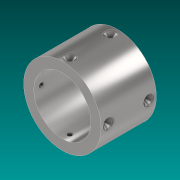
# Autodesk Inventor part: middenGearbox
Saved by Autodesk Inventor 2020.2 (Build 242310000, 310)
## iProperties
Created: 2020-05-14
Part Number: middenGearbox
Material: Stainless Steel
Document SubType Name: Modeling
Designer: Svend
Density: 8 g/cm^3
Appearance: Semi-Polished
Author: Svend
Autodesk Inventor part; units mm, degrees
ref_plane "XY Plane" through (0, 0, 0) normal (0, 0, 1) x (1, 0, 0)
sketch "Sketch1" plane through (0, 0, 0) normal (0, 0, 1) x (1, 0, 0)
  circle A0 centre (0, 0) radius 21
  circle A1 centre (0, 0) radius 15.5
  dimension "d0" = 42
  dimension "d1" = 31
  constraints: 2 centre point, 2 coincident
  measures "d0" diameter of A0
  measures "d1" diameter of A1
extrude "Extrusion1" add sketch "Sketch1" along normal mid plane 30
ref_plane "Work Plane1" through (21, 0, 0) normal (1, 0, 0) x (0, 1, 0)
ref_plane "Work Plane2" through (-21, 0, 0) normal (1, 0, 0) x (0, 1, 0)
ref_plane "Work Plane3" through (0, 21, 0) normal (0, 1, 0) x (-1, 0, 0)
ref_plane "Work Plane4" through (0, -21, 0) normal (0, 1, 0) x (-1, 0, 0)
sketch "Sketch3" plane through (-21, 0, 0) normal (1, 0, 0) x (0, 1, 0)
  line L0 (0, 21) -> (0, -21) projected
  line L1 (21, 15) -> (-21, 15) projected
  line L2 (-21, -15) -> (21, -15) projected
  point P0 (0, 0)
  point P1 (0, -11)
  point P2 (0, 11)
  dimension "d17" = 4
  dimension "d18" = 4
  constraints: 2 point on line
  measures "d17" distance from line of L2 point (0, -11)
  measures "d18" distance from line of L1 point (0, 11)
hole "Hole2" at (-21, 0, -11) at (-21, 0, 11) direction (1, 0, 0) diameter 6 depth 1
sketch "Sketch4" plane through (0, -21, 0) normal (0, 1, 0) x (-1, 0, 0)
  line L0 (21, 15) -> (-21, 15) projected
  line L1 (-21, -15) -> (21, -15) projected
  line L2 (0, -21) -> (0, 21) projected
  point P0 (0, 0)
  point P1 (0, -11)
  point P2 (0, 11)
  dimension "d26" = 4
  dimension "d27" = 4
  constraints: 2 point on line
  measures "d26" distance from line of L0 point (0, 11)
  measures "d27" distance from line of L1 point (0, -11)
hole "Hole3" at (0, -21, -11) at (0, -21, 11) direction (0, 1, 0) diameter 6 depth 1
sketch "Sketch5" plane through (21, 0, 0) normal (1, 0, 0) x (0, 1, 0)
  circle A0 centre (0, -11) radius 3 projected
  circle A1 centre (0, 11) radius 3 projected
  line L0 (-21, -15) -> (21, -15) projected
  point P0 (0, 0)
extrude "Extrusion2" cut sketch "Sketch5" against normal blind 1
sketch "Sketch6" plane through (0, 21, 0) normal (0, 1, 0) x (-1, 0, 0)
  circle A0 centre (0, -11) radius 3 projected
  circle A1 centre (0, 11) radius 3 projected
  point P0 (0, 0)
extrude "Extrusion3" cut sketch "Sketch6" against normal blind 1
sketch "Sketch7" plane through (0, 20, 11) normal (0, 1, 0) x (1, 0, 0)
  circle A0 centre (0, 0) radius 3 projected
  circle A1 centre (0, 22) radius 3 projected
  point P0 (0, 11)
  constraints: 2 coincident
hole "Hole4" at (0, 20, 11) at (0, 20, -11) direction (0, -1, 0) diameter 2.459 depth 8.8 countersink diameter 6 countersink angle 90 thread size "M3x0.5" class "6H" standard "ISO Metric profile"
sketch "Sketch8" plane through (20, 0, -11) normal (1, 0, 0) x (0, 0, -1)
  circle A0 centre (0, 0) radius 3 projected
  circle A1 centre (-22, 0) radius 3 projected
  point P0 (-11, 0)
  constraints: 2 coincident
hole "Hole5" at (20, 0, -11) at (20, 0, 11) direction (-1, 0, 0) diameter 2.459 depth 8.8 countersink diameter 6 countersink angle 90 thread size "M3x0.5" class "6H" standard "ISO Metric profile"
sketch "Sketch9" plane through (0, -20, 11) normal (0, -1, 0) x (1, 0, 0)
  circle A0 centre (0, 0) radius 3 projected
  circle A1 centre (0, -22) radius 3 projected
  point P0 (0, -11)
  constraints: 2 coincident
hole "Hole6" at (0, -20, 11) at (0, -20, -11) direction (0, 1, 0) diameter 2.459 depth 8.8 countersink diameter 6 countersink angle 90 thread size "M3x0.5" class "6H" standard "ISO Metric profile"
sketch "Sketch10" plane through (-20, 0, 11) normal (-1, 0, 0) x (0, 0, 1)
  circle A0 centre (0, 0) radius 3 projected
  circle A1 centre (-22, 0) radius 3 projected
  point P0 (-11, 0)
  constraints: 2 coincident
hole "Hole7" at (-20, 0, 11) at (-20, 0, -11) direction (1, 0, 0) diameter 2.459 depth 8.8 countersink diameter 6 countersink angle 90 thread size "M3x0.5" class "6H" standard "ISO Metric profile"
equation "\"d17\" = d18"
equation "\"d27\" = d26"
body "Solid1"
